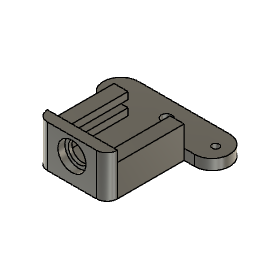
canon_stand_v2 (Autodesk Fusion 360 design; units mm, degrees)
Autodesk Fusion 360 part; units mm, degrees
sketch "Sketch1" plane through (0, 0, 0) normal (0, 0, 1) x (1, 0, 0)
  line L0 (0, 0) -> (35, 0)
  line L1 (35, 0) -> (35, 35)
  line L2 (35, 35) -> (0, 35)
  line L3 (0, 35) -> (0, 0)
  dimension "d1" = 35
  dimension "d2" = 35
  constraint horizontal L0
  constraint vertical L1
  constraint horizontal L2
  constraint vertical L3
  constraint coincident L0.start L3.end
  measures "d1" distance of L0.start L0.end
  measures "d2" distance of L0.start L2.end
extrude "Extrude1" add sketch "Sketch1" along normal blind 3
sketch "Sketch2" plane through (0, 0, 3) normal (0, 0, 1) x (-1, 0, 0)
  line L0 (0, -35) -> (0, 0)
  line L1 (0, 0) -> (-35, 0)
  line L2 (-35, 0) -> (-35, -35)
  line L3 (-35, -35) -> (0, -35)
  line L4 (-10, -35) -> (-35, -35)
  line L5 (-35, -35) -> (-35, -17.5)
  line L6 (-35, -17.5) -> (-10, -17.5)
  line L7 (-10, -17.5) -> (-10, -35)
  dimension "d5" = 25
  dimension "d6" = 17.5
  constraint horizontal L4
  constraint vertical L5
  constraint horizontal L6
  constraint vertical L7
  constraint coincident L2 L5.end
  constraint coincident L3 L4.start
  measures "d5" distance of L4.start L2.end
  measures "d6" distance of L2.end L5.end
extrude "Extrude2" cut sketch "Sketch2" against normal blind 3 contours L2 L3 L4 L5 L6 L7
sketch "Sketch6" plane through (0, 0, 3) normal (0, 0, 1) x (-1, 0, 0)
  line L0 (-35, -17.5) -> (-10, -17.5)
  line L1 (-10, -17.5) -> (-10, -35)
  line L2 (-10, -35) -> (0, -35)
  line L3 (0, -35) -> (0, 0)
  line L4 (0, 0) -> (-35, 0)
  line L5 (-35, 0) -> (-35, -17.5)
  line L6 (-10, -17.5) -> (-14, -17.5)
  line L7 (-14, -17.5) -> (-14, 0)
  line L8 (-14, 0) -> (-10, 0)
  line L9 (-10, 0) -> (-10, -17.5)
  dimension "d23" = 4
  dimension "d24" = 17.5
  constraint horizontal L6
  constraint vertical L7
  constraint horizontal L8
  constraint vertical L9
  constraint coincident L0.end L1.start
  measures "d23" distance of L0.end L6.end
  measures "d24" distance of L0.end L8.end
extrude "Extrude6" add sketch "Sketch6" along normal blind 6 contours L0 L4 L6 L7 L8 L9
extrude "Extrude7" cut 1 faces at (35, 5.8333, 1) along direction (-1, 0, 0) blind 5
sketch "Sketch7" plane through (0, 0, 3) normal (0, 0, 1) x (-1, 0, 0)
  line L0 (-30, 0) -> (-30, -17.5)
  line L1 (-30, -17.5) -> (-14, -17.5)
  line L2 (-14, -17.5) -> (-14, 0)
  line L3 (-14, 0) -> (-30, 0)
  line L4 (-30, -17.5) -> (-26, -17.5)
  line L5 (-26, -17.5) -> (-26, 0)
  line L6 (-26, 0) -> (-30, 0)
  line L7 (-30, 0) -> (-30, -17.5)
  dimension "d29" = 4
  dimension "d30" = 17.5
  constraint horizontal L4
  constraint vertical L5
  constraint horizontal L6
  constraint vertical L7
  constraint coincident L0.end L1.start
  measures "d29" distance of L0.end L4.end
  measures "d30" distance of L0.end L0.start
extrude "Extrude8" add sketch "Sketch7" along normal blind 6 contours L0 L1 L3 L4 L5 L6 L7
extrude "Extrude9" add 1 faces at (28.6667, 17.5, 4) along direction (0, 1, 0) blind 3.5
sketch "Sketch8" plane through (14, 0, 0) normal (1, 0, 0) x (0, 1, 0)
  line L0 (0, 3) -> (21, 3)
  line L1 (21, 3) -> (21, 9)
  line L2 (21, 9) -> (0, 9)
  line L3 (0, 9) -> (0, 3)
  line L4 (0, 7) -> (21, 7)
  line L5 (21, 7) -> (21, 5)
  line L6 (21, 5) -> (0, 5)
  line L7 (0, 5) -> (0, 7)
  dimension "d35" = 2
  dimension "d36" = 2
  constraint horizontal L4
  constraint vertical L5
  constraint horizontal L6
  constraint vertical L7
  constraint coincident L3 L4.start
  measures "d35" distance of L4.start L6.end
  measures "d36" distance of L2 L4
extrude "Extrude10" cut sketch "Sketch8" against normal blind 2 contours L1 L3 L4 L5 L6 L7
sketch "Sketch9" plane through (26, 0, 0) normal (-1, 0, 0) x (0, -1, 0)
  line L0 (-21, 3) -> (0, 3)
  line L1 (0, 3) -> (0, 9)
  line L2 (0, 9) -> (-21, 9)
  line L3 (-21, 9) -> (-21, 3)
  line L4 (-21, 7) -> (0, 7)
  line L5 (0, 7) -> (0, 5)
  line L6 (0, 5) -> (-21, 5)
  line L7 (-21, 5) -> (-21, 7)
  dimension "d39" = 2
  dimension "d40" = 2
  constraint horizontal L4
  constraint vertical L5
  constraint horizontal L6
  constraint vertical L7
  constraint coincident L3 L4.start
  measures "d39" distance of L4.start L6.end
  measures "d40" distance of L2 L4
extrude "Extrude11" cut sketch "Sketch9" against normal blind 2 contours L1 L3 L4 L5 L6 L7
sketch "Sketch10" plane through (0, 0, 5) normal (0, 0, 1) x (-1, 0, 0)
  line L0 (-26, -21) -> (-26, 0)
  line L1 (-26, 0) -> (-28, 0)
  line L2 (-28, 0) -> (-28, -21)
  line L3 (-28, -21) -> (-26, -21)
  line L4 (-26, 0) -> (-28, 0)
  line L5 (-28, 0) -> (-28, -2)
  line L6 (-28, -2) -> (-26, -2)
  line L7 (-26, -2) -> (-26, 0)
  dimension "d43" = 2
  dimension "d44" = 2
  constraint horizontal L4
  constraint vertical L5
  constraint horizontal L6
  constraint vertical L7
  constraint coincident L0.end L1.start
  measures "d43" distance of L0.end L1.end
  measures "d44" distance of L0.end L6.end
extrude "Extrude12" add sketch "Sketch10" along normal blind 2 contours L0 L1 L2 L4 L5 L6 L7
sketch "Sketch11" plane through (0, 0, 5) normal (0, 0, 1) x (-1, 0, 0)
  line L0 (-14, 0) -> (-14, -21)
  line L1 (-14, -21) -> (-12, -21)
  line L2 (-12, -21) -> (-12, 0)
  line L3 (-12, 0) -> (-14, 0)
  line L4 (-14, 0) -> (-12, 0)
  line L5 (-12, 0) -> (-12, -2)
  line L6 (-12, -2) -> (-14, -2)
  line L7 (-14, -2) -> (-14, 0)
  dimension "d47" = 2
  dimension "d48" = 2
  constraint horizontal L4
  constraint vertical L5
  constraint horizontal L6
  constraint vertical L7
  constraint coincident L0.start L3.end
  measures "d47" distance of L0.start L2.end
  measures "d48" distance of L0.start L6.end
extrude "Extrude13" add sketch "Sketch11" along normal blind 2 contours L0 L2 L3 L4 L5 L6 L7
sketch "Sketch14" plane through (0, 21, 0) normal (0, 1, 0) x (-1, 0, 0)
  line L0 (-26, 5) -> (-28, 5)
  line L1 (-28, 5) -> (-28, 7)
  line L2 (-28, 7) -> (-26, 7)
  line L3 (-26, 7) -> (-26, 9)
  line L4 (-26, 9) -> (-30, 9)
  line L5 (-30, 9) -> (-30, 0)
  line L6 (-30, 0) -> (-10, 0)
  line L7 (-10, 0) -> (-10, 3)
  line L8 (-10, 3) -> (-10, 9)
  line L9 (-10, 9) -> (-14, 9)
  line L10 (-14, 9) -> (-14, 7)
  line L11 (-14, 7) -> (-12, 7)
  line L12 (-12, 7) -> (-12, 5)
  line L13 (-12, 5) -> (-14, 5)
  line L14 (-14, 5) -> (-14, 3)
  line L15 (-14, 3) -> (-26, 3)
  line L16 (-26, 3) -> (-26, 5)
  line L17 (-10, 3) -> (-30, 3)
  line L18 (-30, 3) -> (-30, 0)
  line L19 (-30, 0) -> (-10, 0)
  line L20 (-10, 0) -> (-10, 3)
  dimension "d61" = 20
  constraint horizontal L17
  constraint vertical L18
  constraint horizontal L19
  constraint vertical L20
  constraint coincident L7.end L8.start
  measures "d61" distance of L7.end L17.end
extrude "Extrude17" add sketch "Sketch14" along normal blind 10 contours L5 L6 L7 L15 L17 L18 L19 L20
extrude "Extrude18" cut 1 faces at (0, 23.3333, 1) along direction (1, 0, 0) blind 10
sketch "Sketch15" plane through (10, 0, 0) normal (-1, 0, 0) x (0, -1, 0)
  line L0 (0, 0) -> (0, 9)
  line L1 (0, 9) -> (-21, 9)
  line L2 (-21, 9) -> (-21, 3)
  line L3 (-21, 3) -> (-31, 3)
  line L4 (-31, 3) -> (-31, 0)
  line L5 (-31, 0) -> (0, 0)
  line L6 (-21, 3) -> (-31, 3)
  line L7 (-31, 3) -> (-31, 0)
  line L8 (-31, 0) -> (-21, 0)
  line L9 (-21, 0) -> (-21, 3)
  constraint horizontal L6
  constraint vertical L7
  constraint horizontal L8
  constraint vertical L9
  constraint coincident L2.end L3.start
extrude "Extrude19" add sketch "Sketch15" along normal blind 8 contours L3 L4 L5 L6 L7 L8 L9
sketch "Sketch16" plane through (30, 0, 0) normal (1, 0, 0) x (0, 1, 0)
  line L0 (21, 9) -> (0, 9)
  line L1 (0, 9) -> (0, 0)
  line L2 (0, 0) -> (31, 0)
  line L3 (31, 0) -> (31, 3)
  line L4 (31, 3) -> (21, 3)
  line L5 (21, 3) -> (21, 9)
  line L6 (21, 3) -> (31, 3)
  line L7 (31, 3) -> (31, 0)
  line L8 (31, 0) -> (21, 0)
  line L9 (21, 0) -> (21, 3)
  dimension "d68" = 10
  constraint horizontal L6
  constraint vertical L7
  constraint horizontal L8
  constraint vertical L9
  constraint coincident L4.end L5.start
  measures "d68" distance of L4.end L3.end
extrude "Extrude20" add sketch "Sketch16" along normal blind 8 contours L2 L3 L4 L6 L7 L8 L9
sketch "Sketch17" plane through (0, 0, 0) normal (0, 0, -1) x (1, 0, 0)
  line L0 (10, 0) -> (10, -21)
  line L1 (10, -21) -> (2, -21)
  line L2 (2, -21) -> (2, -31)
  line L3 (2, -31) -> (38, -31)
  line L4 (38, -31) -> (38, -21)
  line L5 (38, -21) -> (30, -21)
  line L6 (30, -21) -> (30, 0)
  line L7 (30, 0) -> (10, 0)
  circle A0 centre (20, -26) radius 1.5
  dimension "d71" = 3
  dimension "d72" = 5
  dimension "d73" = 10
  measures "d71" diameter of A0
  measures "d72" distance of L3 A0.centre
  measures "d73" distance of L0 A0.centre
extrude "Extrude21" cut sketch "Sketch17" against normal blind 3 contours A0
sketch "Sketch18" plane through (0, 0, 0) normal (0, 0, -1) x (1, 0, 0)
  circle A0 centre (20, -26) radius 1.5
  line L0 (10, 0) -> (10, -21)
  line L1 (10, -21) -> (2, -21)
  line L2 (2, -21) -> (2, -31)
  line L3 (2, -31) -> (38, -31)
  line L4 (38, -31) -> (38, -21)
  line L5 (38, -21) -> (30, -21)
  line L6 (30, -21) -> (30, 0)
  line L7 (30, 0) -> (10, 0)
  circle A1 centre (6, -26) radius 1
  dimension "d76" = 2
  dimension "d77" = 14
  measures "d76" diameter of A1
  measures "d77" distance of A0.centre A1.centre
extrude "Extrude22" cut sketch "Sketch18" against normal blind 3 contours A1
sketch "Sketch19" plane through (0, 0, 0) normal (0, 0, -1) x (1, 0, 0)
  circle A0 centre (6, -26) radius 1
  circle A1 centre (20, -26) radius 1.5
  line L0 (10, 0) -> (10, -21)
  line L1 (10, -21) -> (2, -21)
  line L2 (2, -21) -> (2, -31)
  line L3 (2, -31) -> (38, -31)
  line L4 (38, -31) -> (38, -21)
  line L5 (38, -21) -> (30, -21)
  line L6 (30, -21) -> (30, 0)
  line L7 (30, 0) -> (10, 0)
  circle A2 centre (34, -26) radius 1
  dimension "d80" = 2
  dimension "d81" = 14
  dimension "d82" = 5
  measures "d80" diameter of A2
  measures "d81" distance of A1.centre A2.centre
  measures "d82" distance of L5 A2.centre
extrude "Extrude23" cut sketch "Sketch19" against normal blind 3 contours A2
fillet "Fillet1" radius 5 1 edges at (38, 21, 1.5)
fillet "Fillet2" radius 5 1 edges at (38, 31, 1.5)
fillet "Fillet3" radius 5 1 edges at (2, 31, 1.5)
fillet "Fillet4" radius 5 1 edges at (2, 21, 1.5)
sketch "Sketch20" plane through (0, 0, 3) normal (0, 0, 1) x (-1, 0, 0)
  arc A0 (-7, -31) -> (-7, -21) centre (-7, -26) ccw
  line L0 (-7, -21) -> (-10, -21)
  line L1 (-10, -21) -> (-14, -21)
  line L2 (-14, -21) -> (-14, 0)
  line L3 (-14, 0) -> (-26, 0)
  line L4 (-26, 0) -> (-26, -21)
  line L5 (-26, -21) -> (-30, -21)
  line L6 (-30, -21) -> (-33, -21)
  arc A1 (-33, -21) -> (-33, -31) centre (-33, -26) ccw
  line L7 (-33, -31) -> (-7, -31)
  circle A2 centre (-34, -26) radius 1
  circle A3 centre (-6, -26) radius 1
  circle A4 centre (-20, -26) radius 1.5
  line L8 (-14, 0) -> (-26, 0)
  line L9 (-26, 0) -> (-26, -2)
  line L10 (-26, -2) -> (-14, -2)
  line L11 (-14, -2) -> (-14, 0)
  dimension "d93" = 2
  constraint horizontal L8
  constraint vertical L9
  constraint horizontal L10
  constraint vertical L11
  constraint coincident L2.end L3.start
  measures "d93" distance of L2.end L10.end
extrude "Extrude24" add sketch "Sketch20" along normal blind 6 contours L2 L3 L4 L8 L9 L10 L11
extrude "Extrude25" add 1 faces at (28.6667, 7.6667, 9) along direction (0, 0, 1) blind 3
extrude "Extrude26" add 1 faces at (23.3333, 0, 8) along direction (0, -1, 0) blind 1
sketch "Sketch22" plane through (0, -1, 0) normal (0, -1, 0) x (1, 0, 0)
  line L0 (10, 12) -> (10, 0)
  line L1 (10, 0) -> (30, 0)
  line L2 (30, 0) -> (30, 12)
  line L3 (30, 12) -> (10, 12)
  circle A0 centre (20, 7) radius 4
  dimension "d104" = 8
  dimension "d105" = 5
  dimension "d106" = 10
  measures "d104" diameter of A0
  measures "d105" distance of L3 A0.centre
  measures "d106" distance of L2 A0.centre
extrude "Extrude27" cut sketch "Sketch22" against normal blind 2 contours A0
sketch "Sketch23" plane through (0, 1, 0) normal (0, -1, 0) x (1, 0, 0)
  circle A0 centre (20, 7) radius 4
  circle A1 centre (20, 7) radius 3
  dimension "d109" = 6
  constraint concentric A0 A1
  measures "d109" diameter of A1
extrude "Extrude28" cut sketch "Sketch23" against normal blind 1 contours A1
sketch "Sketch24" plane through (0, 0, 12) normal (0, 0, 1) x (-1, 0, 0)
  line L0 (-30, 1) -> (-30, -21)
  line L1 (-30, -21) -> (-26, -21)
  line L2 (-26, -21) -> (-26, -2)
  line L3 (-26, -2) -> (-14, -2)
  line L4 (-14, -2) -> (-14, -21)
  line L5 (-14, -21) -> (-10, -21)
  line L6 (-10, -21) -> (-10, 1)
  line L7 (-10, 1) -> (-30, 1)
  line L8 (-26, -21) -> (-30, -21)
  line L9 (-30, -21) -> (-30, -2)
  line L10 (-30, -2) -> (-26, -2)
  line L11 (-26, -2) -> (-26, -21)
  constraint horizontal L8
  constraint vertical L9
  constraint horizontal L10
  constraint vertical L11
  constraint coincident L1.end L2.start
extrude "Extrude29" cut sketch "Sketch24" against normal blind 3 contours L0 L1 L2 L8 L9 L10 L11
sketch "Sketch25" plane through (0, 0, 12) normal (0, 0, 1) x (-1, 0, 0)
  line L0 (-30, -2) -> (-14, -2)
  line L1 (-14, -2) -> (-14, -21)
  line L2 (-14, -21) -> (-10, -21)
  line L3 (-10, -21) -> (-10, 1)
  line L4 (-10, 1) -> (-30, 1)
  line L5 (-30, 1) -> (-30, -2)
  line L6 (-10, -21) -> (-14, -21)
  line L7 (-14, -21) -> (-14, -2)
  line L8 (-14, -2) -> (-10, -2)
  line L9 (-10, -2) -> (-10, -21)
  dimension "d114" = 4
  constraint horizontal L6
  constraint vertical L7
  constraint horizontal L8
  constraint vertical L9
  constraint coincident L2.end L3.start
  measures "d114" distance of L2.end L1.end
extrude "Extrude30" cut sketch "Sketch25" against normal blind 3 contours L1 L2 L3 L6 L7 L8 L9
fillet "Fillet5" radius 3 1 edges at (30, -1, 6)
fillet "Fillet6" radius 3 1 edges at (10, -1, 6)
